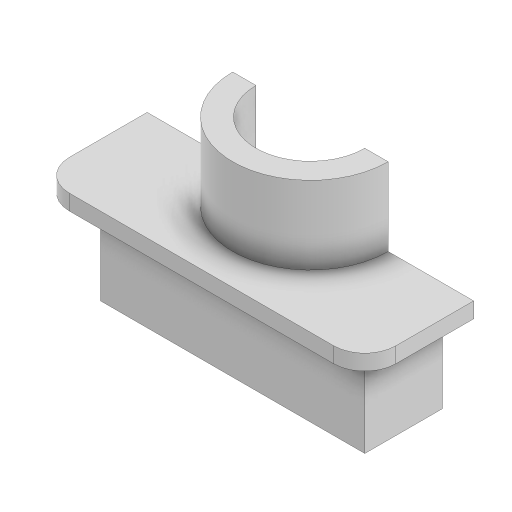
# Autodesk Inventor part: держатель проводной
Saved by Autodesk Inventor 2023.2 (Build 272271000, 271)
## iProperties
Created: 2023-11-25
Part Number: держатель проводной
Material: Типовые
Document SubType Name: Modeling
Designer: matvey
Density: 1 g/cm^3
Appearance: По умолчанию
Author: matvey
Autodesk Inventor part; units mm, degrees
ref_plane "YZ Plane" through (0, 0, 0) normal (1, 0, 0) x (0, 1, 0)
ref_plane "XZ Plane" through (0, 0, 0) normal (0, 1, 0) x (-1, 0, 0)
ref_plane "XY Plane" through (0, 0, 0) normal (0, 0, 1) x (1, 0, 0)
sketch "Эскиз1" plane through (0, 0, 0) normal (0, 0, 1) x (1, 0, 0)
  line L0 (0, 0) -> (-17, 0)
  line L1 (-17, 0) -> (-17, 7)
  line L2 (-17, 7) -> (0, 7)
  line L3 (0, 7) -> (0, 0)
  dimension "d0" = 17
  dimension "d1" = 7
  constraints: 8 end point, 2 parallel, 1 horizontal, 1 perpendicular
  measures "d0" distance between parallel lines of L3 L1
  measures "d1" distance between parallel lines of L0 L2
extrude "Выдавливание1" add sketch "Эскиз1" along normal blind 5
sketch "Эскиз2" plane through (-17, 7, 0) normal (0, 1, 0) x (1, 0, 0)
  line L0 (17, 0) -> (0, 0) projected
  line L1 (0, 0) -> (0, -5) projected
  line L2 (17, -5) -> (0, -5) projected
  line L3 (17, 0) -> (17, -5) projected
  line L4 (17, 0) -> (0, 0) projected
  circle A0 centre (8.5, 0) radius 2.25
  point P0 (6.25, 0)
  point P1 (10.75, 0)
  dimension "d4" = 8.5
  dimension "d5" = 4.5
  constraints: 1 centre point, 1 midpoint
  measures "d4" distance from line of L1 A0.centre
  measures "d5" diameter of A0
extrude "Выдавливание2" cut sketch "Эскиз2" against normal blind 100 contours A0 L0 picked at (8.074, -0.9762)
sketch "Эскиз3" plane through (-17, 7, 5) normal (0, 1, 0) x (1, 0, 0)
  arc A0 (6.25, 5) -> (10.75, 5) centre (8.5, 5) ccw projected
  arc A1 (5, 5) -> (12, 5) centre (8.5, 5) ccw
  arc A2 (3.5, 5) -> (13.5, 5) centre (8.5, 5) ccw
  line L0 (17, 0) -> (0, 0) projected
  line L1 (6.25, 5) -> (0, 5) projected
  line L2 (17, 5) -> (10.75, 5) projected
  dimension "d8" = 7
  constraints: 4 point on circle, 4 point on line, 2 centre point, 2 coincident, 1 tangent
  measures "d8" diameter of A1
extrude "Выдавливание3" add sketch "Эскиз3" along normal blind 5 contours A1 L2 A2 L1
sketch "Эскиз5" plane through (0, 7, 5) normal (0, 1, 0) x (1, 0, 0)
  line L0 (2, 5) -> (-19, 5)
  line L1 (-19, 5) -> (-19, 0)
  line L2 (-17, -2) -> (0, -2)
  line L3 (2, 0) -> (2, 5)
  line L4 (-17, 5) -> (-17, 0) projected
  line L5 (0, 5) -> (0, 0) projected
  line L6 (0, 0) -> (-8.5, 0) projected
  arc A0 (-19, 0) -> (-17, -2) centre (-17, 0) ccw
  arc A1 (0, -2) -> (2, 0) centre (0, 0) ccw
  arc A2 (-13.5, 5) -> (-8.5, 0) centre (-8.5, 5) ccw projected
  line L7 (-13.5, 5) -> (-17, 5) projected
  line L8 (-17, 5) -> (-17, 0) projected
  line L9 (-8.5, 0) -> (-17, 0) projected
  arc A3 (-8.5, 0) -> (-3.5, 5) centre (-8.5, 5) ccw projected
  line L10 (0, 0) -> (-8.5, 0) projected
  line L11 (0, 5) -> (0, 0) projected
  line L12 (0, 5) -> (-3.5, 5) projected
  dimension "d11" = 2
  dimension "d12" = 2
  dimension "d13" = 2
  dimension "d14" = 2
  constraints: 8 end point, 4 point on circle, 4 tangent, 2 centre point, 2 parallel, 1 equal radius, 1 horizontal, 1 perpendicular
  measures "d11" distance between parallel lines of L1 L4
  measures "d12" distance between parallel lines of L3 L5
  measures "d13" distance between parallel lines of L2 L6
  measures "d14" radius of A0
extrude "Выдавливание4" add sketch "Эскиз5" against normal blind 1 contours L3 A1 L2 A0 L1 L0 L4 L9 L6 L5
sketch "Эскиз6" plane through (0, 0, 0) normal (0, 0, -1) x (-1, 0, 0)
  circle A0 centre (3.5, 4) radius 1
  circle A1 centre (13.5, 4) radius 1
  line L0 (8.5, 7.7891) -> (8.5, -0.9569)
  line L1 (6.25, 0) -> (0, 0) projected
  dimension "d17" = 2
  dimension "d18" = 2
  dimension "d19" = 10
  dimension "d20" = 5
  dimension "d21" = 4
  constraints: 2 centre point, 2 end point, 1 horizontal alignment, 1 vertical
  measures "d17" diameter of A0
  measures "d18" diameter of A1
  measures "d19" distance of A1.centre A0.centre
  measures "d20" distance from line of L0 A0.centre
  measures "d21" distance from line of L1 A0.centre
extrude "Выдавливание5" cut sketch "Эскиз6" against normal blind 3
